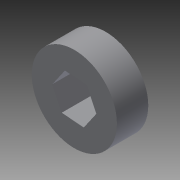
# Autodesk Inventor part: ShaftCollar
Saved by Autodesk Inventor 2013 (Build 170138000, 138)
## iProperties
Created: 2013-01-10
Part Number: ShaftCollar
Material: Generic
Document SubType Name: Modeling
Designer: Naphat
Density: 1 g/cm^3
Mass: 5.1024 g
Surface Area: 23.6515 cm^2
Volume: 5.1024 cm^3
Author: Naphat
Autodesk Inventor part; units mm, degrees
ref_plane "YZ Plane" through (0, 0, 0) normal (1, 0, 0) x (0, 1, 0)
ref_plane "XZ Plane" through (0, 0, 0) normal (0, 1, 0) x (-1, 0, 0)
ref_plane "XY Plane" through (0, 0, 0) normal (0, 0, 1) x (1, 0, 0)
sketch "Sketch1" plane through (0, 0, 0) normal (0, 0, 1) x (1, 0, 0)
  circle A0 centre (-12.936, 0.5481) radius 6.35
  circle A1 centre (-12.936, 0.5481) radius 14.1605
  point P0 (0, 0)
  dimension "d0" = 12.7
  dimension "d1" = 28.321
  constraints: 2 centre point, 1 coincident
  measures "d0" diameter of A0
  measures "d1" diameter of A1
extrude "Extrusion1" add sketch "Sketch1" against normal blind 10.414
sketch "Sketch2" plane through (-12.936, 0.5481, -10.414) normal (0, 0, -1) x (-1, 0, 0)
  circle A0 centre (0, 0) radius 14.1605 projected
  line L0 (3.1289, 6.6404) -> (-4.1863, 6.0299)
  line L1 (3.1289, 6.6404) -> (7.3152, 0.6105)
  line L2 (7.3152, 0.6105) -> (4.1863, -6.0299)
  line L3 (4.1863, -6.0299) -> (-3.1289, -6.6404)
  line L4 (-3.1289, -6.6404) -> (-7.3152, -0.6105)
  line L5 (-7.3152, -0.6105) -> (-4.1863, 6.0299)
  point P0 (-12.936, -0.5481)
  dimension "d5" = 7.3406
  dimension "d6" = 7.3406
  dimension "d7" = 7.3406
  dimension "d8" = 7.3406
  dimension "d9" = 120
  dimension "d10" = 120
  dimension "d11" = 120
  dimension "d12" = 7.3406
  dimension "d13" = 120
  dimension "d14" = 120
  dimension "d15" = 120
  dimension "d16" = 12.7143
  dimension "d17" = 6.3571
  dimension "d18" = 14.6303
  dimension "d19" = 7.3152
  constraints: 12 end point, 1 parallel
  measures "d5" distance of L0.start L0.end
  measures "d6" distance of L0.start L1.end
  measures "d7" distance of L1.end L2.end
  measures "d8" distance of L2.end L3.end
  measures "d9" angle of L0 L1
  measures "d10" angle of L2 L1
  measures "d11" angle of L3 L2
  measures "d12" distance of L3.end L4.end
  measures "d13" angle of L3 L4
  measures "d14" angle of L0 L5
  measures "d15" angle of L4 L5
  measures "d16" distance between parallel lines of L3 L0
  measures "d17" distance from line of L0 A0.centre
  measures "d18" horizontal distance of L1.end L4.end
  measures "d19" horizontal distance of L4.end A0.centre
extrude "Extrusion2" cut sketch "Sketch2" against normal blind 25.4 contours L1 L2 L3 L4 L5 L0
equation "\"d6\" = d5"
equation "\"d7\" = d5"
equation "\"d8\" = d5"
equation "\"d9\" = d10"
equation "\"d12\" = d5"
equation "\"d17\" = 0.5 * d16"
equation "\"d19\" = 0.5 * d18"
body "Solid1"
